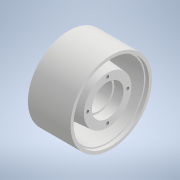
# Autodesk Inventor part: Cilindro Tensor
Saved by Autodesk Inventor 2021 (Build 250183000, 183)
## iProperties
Created: 2020-12-29
Part Number: Cilindro Tensor
Material: Aluminum 6061
Document SubType Name: Modeling
Designer: Miguel Gòmez
Density: 2.7 g/cm^3
Appearance: Aluminum - Flat
Author: Miguel Gòmez
Autodesk Inventor part; units mm, degrees
ref_plane "YZ Plane" through (0, 0, 0) normal (1, 0, 0) x (0, 1, 0)
ref_plane "XZ Plane" through (0, 0, 0) normal (0, 1, 0) x (-1, 0, 0)
ref_plane "XY Plane" through (0, 0, 0) normal (0, 0, 1) x (1, 0, 0)
sketch "Boceto1" plane through (0, 0, 0) normal (0, 0, 1) x (1, 0, 0)
  line L0 (0, 0) -> (0, 40)
  line L1 (0, 40) -> (10, 40)
  line L2 (0, 0) -> (80, 0)
  line L3 (10, 40) -> (10, 0)
  line L4 (10, 0) -> (10, 26)
  line L5 (10, 26) -> (25, 26)
  line L6 (25, 26) -> (25, 0)
  line L7 (25, 0) -> (25, 23)
  line L8 (0, 0) -> (0, 67)
  line L9 (0, 67) -> (70, 67)
  line L10 (0, 67) -> (12, 67) construction
  line L11 (12, 67) -> (12, 0) construction
  line L12 (70, 67) -> (70, 62)
  line L13 (70, 62) -> (64, 62)
  line L14 (70, 62) -> (70, 0)
  line L15 (64, 0) -> (70, 0)
  line L16 (64, 0) -> (70, 0)
  line L17 (64, 62) -> (64, 0)
  line L18 (64, 62) -> (64, 60)
  line L19 (64, 0) -> (64, 39)
  line L20 (64, 60) -> (116.3905, 60) construction
  line L21 (64, 39) -> (116.3905, 39) construction
  line L22 (25, 0) -> (25, 23)
  line L23 (49, 0) -> (49, 23)
  line L24 (49, 23) -> (25, 23)
  line L25 (49, 23) -> (49, 26)
  line L26 (49, 26) -> (64, 26)
  line L27 (64, 39) -> (64, 49.5)
  line L28 (64, 49.5) -> (-5.756, 49.5) construction
  line L29 (12, 49.5) -> (12, 56)
  line L30 (12, 56) -> (12, 43)
  line L31 (12, 56) -> (64, 60)
  line L32 (64, 39) -> (12, 43)
  dimension "d0" = 40
  dimension "d1" = 10
  dimension "d2" = 80
  dimension "d3" = 26
  dimension "d4" = 15
  dimension "d10" = 67
  dimension "d12" = 70
  dimension "d16" = 12
  dimension "d22" = 5
  dimension "d29" = 54
  dimension "d30" = 2
  dimension "d31" = 39
  dimension "d40" = 24
  dimension "d41" = 23
  dimension "d42" = 3
  dimension "d45" = 10.5
  dimension "d46" = 6.5
  dimension "d47" = 13
  constraints: 66 end point, 18 point on line, 10 perpendicular, 6 horizontal, 4 vertical, 2 collinear
  measures "d0" distance of L0.start L0.end
  measures "d1" distance of L0.end L1.end
  measures "d2" distance of L0.start L2.end
  measures "d3" distance of L3.end L4.end
  measures "d4" distance of L4.end L5.end
  measures "d10" distance of L0.start L8.end
  measures "d12" distance of L8.end L9.end
  measures "d16" distance of L8.end L10.end
  measures "d22" distance of L9.end L12.end
  measures "d29" horizontal distance of L13.end L1.end
  measures "d30" distance of L13.end L18.end
  measures "d31" distance of L15.start L19.end
  measures "d40" distance of L6.end L23.start
  measures "d41" distance of L23.start L23.end
  measures "d42" distance of L23.end L25.end
  measures "d45" distance of L19.end L27.end
  measures "d46" distance of L29.start L29.end
  measures "d47" distance of L29.end L30.end
revolve "Revolución1" add sketch "Boceto1" angle 360 about axis through (0, 0, 0) along (1, 0, 0) contours L8 L9 L12 L13 L17 L31 L29 L30 L32 L26 L25 L24 L6 L5 L3 L1
sketch "Boceto4" plane through (10, 0, 0) normal (-1, 0, 0) x (0, 0, 1)
  circle A0 centre (0, 0) radius 33 construction
  circle A1 centre (0, 0) radius 33 construction
  circle A2 centre (0, 0) radius 33 construction
  circle A3 centre (0, 0) radius 33 construction
  point P0 (-33, 0)
  point P1 (0, -33)
  point P2 (33, 0)
  point P3 (0, 33)
  dimension "d61" = 66
  dimension "d64" = 360
  constraints: 2 horizontal alignment, 2 vertical alignment, 1 coincident, 21 other
hole "Agujero2" at (10, 33, 0) at (10, 0, 33) at (10, -33, 0) at (10, 0, -33) direction (1, 0, 0) diameter 4.917 depth 15 tip angle 118 thread size "M6x1" class "6H" standard "ANSI Metric M Profile"
sketch "Boceto5" plane through (64, 0, 0) normal (1, 0, 0) x (0, 0, -1)
  circle A0 centre (0, 0) radius 33 construction
  circle A1 centre (0, 33) radius 2.4585 projected
  circle A2 centre (-33, 0) radius 2.4585 projected
  circle A3 centre (33, 0) radius 2.4585 projected
  circle A4 centre (0, -33) radius 2.4585 projected
  dimension "d73" = 66
  constraints: 5 coincident, 1 centre point
  measures "d73" diameter of A0
hole "Agujero3" at (64, 33, 0) at (64, 0, 33) at (64, 0, -33) at (64, -33, 0) direction (-1, 0, 0) diameter 4.917 depth 18 tip angle 118 thread size "M6x1" class "6H" standard "ANSI Metric M Profile"
